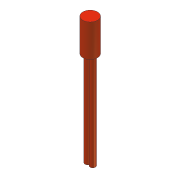
# Autodesk Inventor part: thermistor_batteries
Saved by Autodesk Inventor 2014 SP1 (Build 180222100, 222)
## iProperties
Created: 2013-07-10
Part Number: thermistor_batteries
Document SubType Name: Modeling
Designer: Robert Davis
Density: 1 g/cm^3
Material: Generic
Appearance: Default
Author: Robert Davis
Autodesk Inventor part; units mm, degrees
ref_plane "YZ Plane" through (0, 0, 0) normal (1, 0, 0) x (0, 1, 0)
ref_plane "XZ Plane" through (0, 0, 0) normal (0, 1, 0) x (-1, 0, 0)
ref_plane "XY Plane" through (0, 0, 0) normal (0, 0, 1) x (1, 0, 0)
sketch "Sketch1" plane through (0, 0, 0) normal (0, 0, 1) x (1, 0, 0)
  circle A0 centre (0, 0) radius 1.143
  dimension "d0" = 2.286
  constraints: 1 centre point, 1 coincident
  measures "d0" diameter of A0
extrude "Extrusion1" add sketch "Sketch1" along normal mid plane 5.08
sketch "Sketch2" plane through (0, 0, -2.54) normal (0, 0, -1) x (-1, 0, 0)
  circle A0 centre (0, 0) radius 1.143 projected
  circle A1 centre (-0.4064, 0) radius 0.4064
  circle A2 centre (0.4064, 0) radius 0.4064
  line L0 (-0.828, 0) -> (0.828, 0) construction
  dimension "d3" = 0.8128
  constraints: 2 end point, 2 horizontal alignment, 2 point on line, 1 coincident, 1 horizontal, 1 midpoint, 4 other
extrude "Extrusion2" add sketch "Sketch2" along normal blind 15 contours A1 | A2
body "Solid1"
